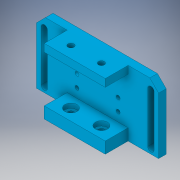
# Autodesk Inventor part: КВ33.044.702 - Стойка натягивающих роликов оси Y
Saved by Autodesk Inventor 2019 (Build 230136000, 136)
## iProperties
Created: 2019-08-19
Part Number: КВ33.044.702 - Стойка натягивающих роликов оси Y
Material: Пластик АБС
Document SubType Name: Modeling
Designer: Петров Иван
Density: 1.06 g/cm^3
Appearance: Небесно-голубой — нейтральный
Author: Петров Иван
Autodesk Inventor part; units mm, degrees
ref_plane "YZ Plane" through (0, 0, 0) normal (1, 0, 0) x (0, 1, 0)
ref_plane "XZ Plane" through (0, 0, 0) normal (0, 1, 0) x (-1, 0, 0)
ref_plane "XY Plane" through (0, 0, 0) normal (0, 0, 1) x (1, 0, 0)
sketch "Эскиз1" plane through (0, 0, 0) normal (0, 0, 1) x (1, 0, 0)
  arc A0 (50, 23.4174) -> (30, 23.4174) centre (40, 28) ccw
  line L0 (0, 37.25) -> (5.75, 43)
  line L1 (0, 0) -> (0, 37.25)
  line L2 (80, 0) -> (0, 0)
  line L3 (80, 0) -> (80, 37.25)
  line L4 (74.25, 43) -> (80, 37.25)
  line L5 (5.75, 43) -> (74.25, 43)
  circle A1 centre (40, 28) radius 2
  arc A2 (2.9, 3.4608) -> (7.1, 3.4608) centre (5, 3.4608) ccw
  line L6 (2.9, 3.4608) -> (2.9, 36.5392)
  arc A3 (7.1, 36.5392) -> (2.9, 36.5392) centre (5, 36.5392) ccw
  line L7 (7.1, 36.5392) -> (7.1, 3.4608)
  arc A4 (77.1, 36.5392) -> (72.9, 36.5392) centre (75, 36.5392) ccw
  line L8 (77.1, 36.5392) -> (77.1, 3.4608)
  arc A5 (72.9, 3.4608) -> (77.1, 3.4608) centre (75, 3.4608) ccw
  line L9 (72.9, 3.4608) -> (72.9, 36.5392)
  point P0 (40, -34)
  constraints: 20 end point, 10 point on circle, 6 centre point
extrude "Выдавливание1" add sketch "Эскиз1" along normal blind 5
sketch "Эскиз2" plane through (0, 0, 5) normal (0, 0, 1) x (1, 0, 0)
  line L0 (60, 0) -> (60, 7.5)
  line L1 (60, 7.5) -> (20, 7.5)
  line L2 (20, 7.5) -> (20, 0)
  line L3 (0, 0) -> (80, 0) projected
  line L4 (40, 0) -> (60, 7.5) construction
  line L5 (40, 0) -> (20, 7.5) construction
  line L6 (60, 0) -> (20, 0)
  dimension "d2" = 40
  constraints: 12 end point, 2 point on line, 1 midpoint, 1 parallel
  measures "d2" distance of L1.end L0.end
extrude "Выдавливание2" add sketch "Эскиз2" along normal blind 15
sketch "Эскиз3" plane through (20, 7.5, 5) normal (0, 1, 0) x (1, 0, 0)
  line L0 (0, 0) -> (0, -15) projected
  line L1 (0, -7.5) -> (40, -7.5)
  line L2 (40, 0) -> (40, -15) projected
  line L3 (20, -7.5) -> (20, -15)
  line L4 (20, -7.5) -> (20, 0)
  circle A0 centre (10, -7.5) radius 1.95
  circle A1 centre (30, -7.5) radius 1.95
  point P0 (-20, 5)
  dimension "d6" = 3.9
  constraints: 6 end point, 3 midpoint, 2 centre point, 2 vertical, 1 point on line, 1 symmetric about line, 1 other
  measures "d6" diameter of A0
extrude "Выдавливание3" cut sketch "Эскиз3" against normal blind 15
sketch "Эскиз4" plane through (20, 7.5, 5) normal (0, 1, 0) x (1, 0, 0)
  circle A0 centre (10, -7.5) radius 1.95 projected
  circle A1 centre (10, -7.5) radius 4
  circle A2 centre (30, -7.5) radius 1.95 projected
  circle A3 centre (30, -7.5) radius 4
  point P0 (-20, 5)
  dimension "d9" = 8
  dimension "d10" = 8
  constraints: 2 centre point, 2 coincident
  measures "d9" diameter of A1
  measures "d10" diameter of A3
extrude "Выдавливание4" cut sketch "Эскиз4" against normal blind 3
sketch "Эскиз5" plane through (0, 0, 0) normal (0, 0, -1) x (-1, 0, 0)
  arc A0 (-30, 23.4174) -> (-50, 23.4174) centre (-40, 28) ccw
  line L0 (-30, 23.4174) -> (-30, 0)
  line L1 (-11.1, 0) -> (-30, 0)
  line L2 (-11.1, 0) -> (-11.1, 37.25)
  line L3 (-13.85, 40) -> (-11.1, 37.25)
  line L4 (-66.15, 40) -> (-13.85, 40)
  line L5 (-68.9, 37.25) -> (-66.15, 40)
  line L6 (-68.9, 0) -> (-68.9, 37.25)
  line L7 (-50, 0) -> (-68.9, 0)
  line L8 (-50, 0) -> (-50, 23.4174)
  circle A1 centre (-26.5, 13.5) radius 1.3
  circle A2 centre (-53.5, 21.5) radius 1.3
  circle A3 centre (-53.5, 5.5) radius 1.3
  circle A4 centre (-53.5, 13.5) radius 1.3
  circle A5 centre (-26.5, 5.5) radius 1.3
  circle A6 centre (-26.5, 21.5) radius 1.3
  circle A7 centre (-40, 28) radius 2 projected
  circle A8 centre (-40, 28) radius 2
  point P0 (0, 0)
  point P1 (28.9, -34)
  constraints: 18 end point, 8 centre point, 2 point on circle, 1 coincident
extrude "Выдавливание5" cut sketch "Эскиз5" against normal through all contours A1 | A2 | A4 | A6
sketch "Эскиз9" plane through (5.75, 43, 0) normal (0, 1, 0) x (1, 0, 0)
  line L0 (54.25, -20) -> (14.25, -20) projected
  line L1 (14.25, -5) -> (54.25, -5) projected
  line L2 (54.25, -20) -> (14.25, -20)
  line L3 (14.25, -20) -> (14.25, -5)
  line L4 (14.25, -5) -> (54.25, -5)
  line L5 (54.25, -5) -> (54.25, -20)
  circle A0 centre (44.25, -12.5) radius 1.95 projected
  circle A1 centre (44.25, -12.5) radius 1.95
  circle A2 centre (24.25, -12.5) radius 1.95 projected
  circle A3 centre (24.25, -12.5) radius 1.95
  point P0 (-5.75, 0)
  constraints: 8 end point, 2 centre point, 2 coincident, 2 parallel, 1 horizontal, 1 perpendicular
extrude "Выдавливание8" add sketch "Эскиз9" against normal blind 5
